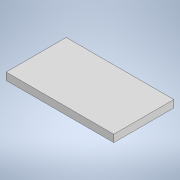
# Autodesk Inventor part: Model1
Saved by Autodesk Inventor 2020.3 (Build 243373000, 373)
## iProperties
Created: 2021-03-22
Part Number: Model1
Material: Generic
Document SubType Name: Modeling
Designer: alexo
Density: 1 g/cm^3
Appearance: Default
Author: alexo
Autodesk Inventor part; units mm, degrees
ref_plane "YZ Plane" through (0, 0, 0) normal (1, 0, 0) x (0, 1, 0)
ref_plane "XZ Plane" through (0, 0, 0) normal (0, 1, 0) x (-1, 0, 0)
ref_plane "XY Plane" through (0, 0, 0) normal (0, 0, 1) x (1, 0, 0)
sketch "Sketch1" plane through (0, 0, 0) normal (0, 1, 0) x (-1, 0, 0)
  line L0 (-125.5, -70) -> (125.5, -70)
  line L1 (125.5, -70) -> (125.5, 70)
  line L2 (125.5, 70) -> (-125.5, 70)
  line L3 (-125.5, 70) -> (-125.5, -70)
  line L4 (-125.5, -70) -> (125.5, 70) construction
  line L5 (125.5, -70) -> (-125.5, 70) construction
  point P0 (0, 0)
  dimension "d0" = 140
  dimension "d1" = 251
  constraints: 12 end point, 2 midpoint, 2 parallel, 1 horizontal, 1 perpendicular
  measures "d0" distance of L0.end L1.end
  measures "d1" distance of L1.end L2.end
extrude "Extrusion1" add sketch "Sketch1" along normal blind 17
body "Solid1"
